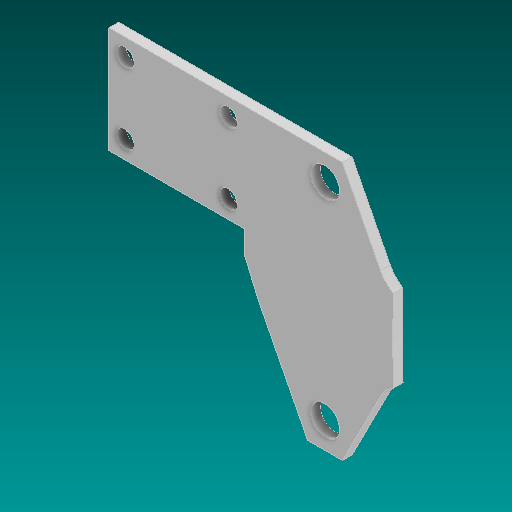
# Autodesk Inventor part: Part22
Saved by Autodesk Inventor 2020 (Build 240168000, 168)
## iProperties
Created: 2022-11-16
Part Number: Part22
Material: 一般
Document SubType Name: Modeling
Designer: Administrator
Density: 1 g/cm^3
Appearance: 既定
Author: Administrator
Autodesk Inventor part; units mm, degrees
ref_plane "YZ Plane" through (0, 0, 0) normal (1, 0, 0) x (0, 1, 0)
ref_plane "XZ Plane" through (0, 0, 0) normal (0, 1, 0) x (-1, 0, 0)
ref_plane "XY Plane" through (0, 0, 0) normal (0, 0, 1) x (1, 0, 0)
sketch "スケッチ1" plane through (0, 0, 0) normal (0, 0, 1) x (1, 0, 0)
  circle A0 centre (5, 0) radius 2.75 projected
  line L0 (14, -5.5) -> (14, 5.5) projected
  line L1 (0, 5.5) -> (14, 5.5) projected
  line L2 (0, -5.5) -> (0, 5.5) projected
  line L3 (14, -5.5) -> (0, -5.5) projected
  circle A1 centre (5, 22) radius 2.75 projected
  line L4 (14, 16.5) -> (14, 27.5) projected
  line L5 (0, 27.5) -> (14, 27.5) projected
  line L6 (0, 16.5) -> (0, 27.5) projected
  line L7 (14, 16.5) -> (0, 16.5) projected
  circle A2 centre (37, 22) radius 2.75 projected
  line L8 (42, 16.5) -> (42, 27.5) projected
  line L9 (28, 27.5) -> (42, 27.5) projected
  line L10 (28, 16.5) -> (28, 27.5) projected
  line L11 (42, 16.5) -> (28, 16.5) projected
  circle A3 centre (37, 0) radius 2.75 projected
  line L12 (42, -5.5) -> (42, 5.5) projected
  line L13 (28, 5.5) -> (42, 5.5) projected
  line L14 (28, -5.5) -> (28, 5.5) projected
  line L15 (42, -5.5) -> (28, -5.5) projected
  line L16 (0, 27.5) -> (90, 27.5)
  line L17 (0, -5.5) -> (0, 27.5)
  line L18 (68.5171, 27.5) -> (108.5171, 27.5) construction
  line L19 (0, 27.5) -> (0, -12.5)
  line L20 (42, -12.5) -> (67, -12.5)
  circle A4 centre (67, -12.5) radius 15
  line L21 (83.6366, -30.4945) -> (83.6366, -28.0767) projected
  line L22 (72.4, -52.5) -> (83.6366, -30.4945) projected
  line L23 (61.6, -52.5) -> (72.4, -52.5) projected
  line L24 (46.516, -22.9597) -> (61.6, -52.5) projected
  arc A5 (46.516, -2.0403) -> (46.516, -22.9597) centre (67, -12.5) ccw projected
  line L25 (61.6, 27.5) -> (46.516, -2.0403) projected
  line L26 (72.4, 27.5) -> (61.6, 27.5) projected
  line L27 (84.2198, 4.3523) -> (72.4, 27.5) projected
  arc A6 (84.2198, 4.3523) -> (93.1259, -1.1) centre (93.1259, 8.9) ccw projected
  line L28 (93.1259, -1.1) -> (88.5, -1.1) projected
  line L29 (88.5, -1.1) -> (86.7345, -1.1) projected
  arc A7 (86.7345, -1.1) -> (83.6366, -28.0767) centre (67, -12.5) ccw projected
  circle A8 centre (67, -44.5) radius 4.5 projected
  circle A9 centre (67, 19.5) radius 4.5 projected
  line L30 (86.3708, -1.1) -> (88, -1.1) projected
  line L31 (88, -1.1) -> (88, -11.75) projected
  line L32 (88, -11.75) -> (81.9812, -11.75) projected
  arc A10 (81.9812, -11.75) -> (81.9812, -13.25) centre (67, -12.5) ccw projected
  line L33 (81.9812, -13.25) -> (88, -13.25) projected
  line L34 (88, -13.25) -> (88, -23.9) projected
  line L35 (86.3708, -23.9) -> (88, -23.9) projected
  arc A11 (86.3708, -1.1) -> (86.3708, -23.9) centre (67, -12.5) ccw projected
  line L36 (88, -11.75) -> (88.5171, 27.5)
  line L37 (88, -11.75) -> (88.5171, -52.5)
  line L38 (88.5171, -52.5) -> (61.6, -52.5)
  line L39 (46.516, -22.9597) -> (61.6, -52.5)
  line L40 (0, -5.5) -> (42, -5.5)
  line L41 (46.516, -22.9597) -> (42, -12.5)
  line L42 (42, -5.5) -> (42, -12.5)
  spline S0 degree 3 poles (88.5, -25.0343) (88.1438, -25.2215) (87.7914, -25.4319) (86.8133, -26.1051) (86.2336, -26.6215) (85.1469, -27.8033) (84.6277, -28.5566) (84.2198, -29.3523) knots 3.82265 3.82265 3.82265 3.82265 3.937981 3.937981 4.159447 4.159447 4.451362 4.451362 4.451362 4.451362 projected
  line L43 (84.2198, -29.3523) -> (83.6366, -30.4945) projected
  point P0 (-38, -5.5)
  point P1 (88.1403, -1.1)
  point P2 (88.1577, 0.2214)
  point P3 (44, -12.5)
  point P4 (45.34, -20.2361)
  point P5 (88.1708, -25.2146)
  dimension "d6" = 40
  dimension "d7" = 25
  dimension "d8" = 30
  constraints: 24 end point, 3 collinear, 3 point on line, 2 horizontal, 1 centre point, 1 coincident, 1 midpoint, 1 perpendicular
  measures "d6" distance of L5.start L19.end
  measures "d7" distance of L20.start L20.end
  measures "d8" diameter of A4
extrude "押し出し1" add sketch "スケッチ1" along normal blind 3 contours L3 L2 L1 L0 | L0 L1 L17 L7 L4 L16 L10 L11 L8 L25 A5 L20 L42 L12 L13 L14 L40 | L14 L13 L12 L15 | L6 L5 L4 L7 | L20 A5 L41 | A5 L25 L16 L27 A6 L36 L29 A7 L20 | L20 A7 L21 L22 L23 L24 L41 A5 | A7 L30 A11 L20 | L20 A11 L35 L34 L33 A4 L32 L37 S0 L43 L21 A7 | L9 L8 L11 L10 | A11 L30 L29 L31 L32 A4 L20 | L20 A4 L33 L34 L35 A11 | A4 | L29 L36 L31
